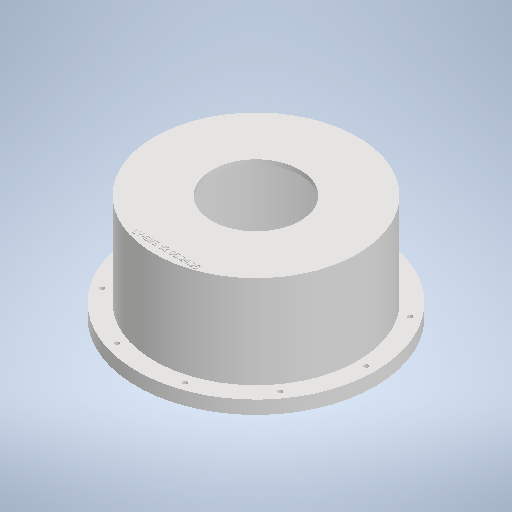
# Autodesk Inventor part: Cylinder Housing
Saved by Autodesk Inventor 2025.2 (Build 292293000, 293)
## iProperties
Created: 2025-06-17
Part Number: Cylinder Housing
Material: Generic
Document SubType Name: Modeling
Designer: mumin
Density: 1 g/cm^3
Appearance: Default
Author: mumin
Autodesk Inventor part; units mm, degrees
note: some values were not read from the file. Chosen so that the rebuilt part matches the saved one: direction of "Hole1".
ref_plane "YZ Plane" through (0, 0, 0) normal (1, 0, 0) x (0, 1, 0)
ref_plane "XZ Plane" through (0, 0, 0) normal (0, 1, 0) x (-1, 0, 0)
ref_plane "XY Plane" through (0, 0, 0) normal (0, 0, 1) x (1, 0, 0)
sketch "Sketch1" plane through (0, 0, 0) normal (0, 1, 0) x (-1, 0, 0)
  circle A0 centre (0, 0) radius 110
  circle A1 centre (0, 0) radius 135
  dimension "d0" = 220
  dimension "d1" = 270
  constraints: 2 centre point, 2 coincident
  measures "d0" diameter of A0
  measures "d1" diameter of A1
extrude "Extrusion1" add sketch "Sketch1" along normal blind 15
sketch "Sketch2" plane through (0, 15, 0) normal (0, 1, 0) x (1, 0, 0)
  circle A0 centre (0, 0) radius 110 projected
  circle A1 centre (0, 0) radius 115
  dimension "d4" = 230
  constraints: 1 centre point, 1 coincident
  measures "d4" diameter of A1
extrude "Extrusion2" add sketch "Sketch2" along normal blind 105
sketch "Sketch3" plane through (0, 120, 0) normal (0, 1, 0) x (1, 0, 0)
  circle A0 centre (0, 0) radius 115 projected
extrude "Extrusion3" add sketch "Sketch3" against normal blind 5
sketch "Sketch4" plane through (0, 120, 0) normal (0, 1, 0) x (1, 0, 0)
  point P0 (0, 0)
  point P1 (0, 0)
  constraints: 1 coincident
hole "Hole1" at (0, 120, 0) direction (0, -1, 0) diameter 100 depth 5
sketch "Sketch5" plane through (0, 15, 0) normal (0, 1, 0) x (1, 0, 0)
  line L0 (-189, 0) -> (189, 0) projected
  point P0 (0, 0)
  point P1 (-125, 0)
  dimension "d23" = 125
  constraints: 1 point on line
  measures "d23" distance of point (0, 0) point (-125, 0)
hole "Hole2" at (-125, 15, 0) direction (0, -1, 0) diameter 5.2 end through all
pattern_circular "Circular Pattern1" count 10 over 360 about axis through (0, -10, 0) along (0, 1, 0) of "Hole2"
sketch "Sketch6" plane through (0, 120, 0) normal (0, 1, 0) x (1, 0, 0)
  line L0 (-34.2404, -100.9913) -> (41.5143, -100.9913) construction
  line L1 (41.5143, -100.9913) -> (41.5143, -112.0132) construction
  line L2 (41.5143, -112.0132) -> (-34.2404, -112.0132) construction
  line L3 (-34.2404, -112.0132) -> (-34.2404, -100.9913) construction
  line L4 (-30.1561, -107.1178) -> (-33.6326, -107.1178)
  line L5 (-33.6326, -107.1178) -> (-33.6326, -101.1178)
  line L6 (-33.6326, -101.1178) -> (-32.8352, -101.1178)
  line L7 (-32.8352, -101.1178) -> (-32.8352, -106.4079)
  line L8 (-32.8352, -106.4079) -> (-30.1561, -106.4079)
  line L9 (-30.1561, -106.4079) -> (-30.1561, -107.1178)
  line L10 (-25.1772, -101.1178) -> (-27.2437, -107.1178)
  line L11 (-27.2437, -107.1178) -> (-28.1043, -107.1178)
  line L12 (-28.1043, -107.1178) -> (-30.1707, -101.1178)
  line L13 (-30.1707, -101.1178) -> (-29.315, -101.1178)
  line L14 (-29.315, -101.1178) -> (-27.6521, -106.1016)
  line L15 (-27.6521, -106.1016) -> (-25.9892, -101.1178)
  line L16 (-25.9892, -101.1178) -> (-25.1772, -101.1178)
  line L17 (-22.5759, -104.8568) -> (-24.8466, -104.8568)
  line L18 (-24.8466, -104.8568) -> (-24.8466, -104.1275)
  line L19 (-24.8466, -104.1275) -> (-22.5759, -104.1275)
  line L20 (-22.5759, -104.1275) -> (-22.5759, -104.8568)
  spline S0 degree 2 poles (-19.0945, -107.2345) (-19.7315, -107.2345) (-20.7866, -106.8455) (-21.1659, -106.4516) knots 0 0 0 1 2 2 2
  spline S1 degree 2 poles (-21.1659, -106.4516) (-21.5451, -106.0529) (-21.9487, -104.8763) (-21.9487, -104.1129) knots 0 0 0 1 2 2 2
  spline S2 degree 2 poles (-21.9487, -104.1129) (-21.9487, -103.3884) (-21.5402, -102.2409) (-21.161, -101.8325) knots 0 0 0 1 2 2 2
  spline S3 degree 2 poles (-21.161, -101.8325) (-20.7963, -101.4387) (-19.7266, -101.0108) (-19.0897, -101.0108) knots 0 0 0 1 2 2 2
  spline S4 degree 2 poles (-19.0897, -101.0108) (-18.7834, -101.0108) (-18.2291, -101.0983) (-17.9762, -101.1761) knots 0 0 0 1 2 2 2
  spline S5 degree 2 poles (-17.9762, -101.1761) (-17.772, -101.2345) (-17.2761, -101.4484) (-17.1253, -101.5262) knots 0 0 0 1 2 2 2
  line L21 (-17.1253, -101.5262) -> (-17.1253, -102.4889)
  line L22 (-17.1253, -102.4889) -> (-17.1934, -102.4889)
  spline S6 degree 2 poles (-17.1934, -102.4889) (-17.3441, -102.3576) (-17.6602, -102.1194) (-17.9519, -101.9832) knots 0 0 0 1 2 2 2
  spline S7 degree 2 poles (-17.9519, -101.9832) (-18.195, -101.8617) (-18.8223, -101.7012) (-19.1821, -101.7012) knots 0 0 0 1 2 2 2
  spline S8 degree 2 poles (-19.1821, -101.7012) (-20.0475, -101.7012) (-21.1172, -103.0043) (-21.1172, -104.0886) knots 0 0 0 1 2 2 2
  spline S9 degree 2 poles (-21.1172, -104.0886) (-21.1172, -104.6915) (-20.8352, -105.5959) (-20.5678, -105.9071) knots 0 0 0 1 2 2 2
  spline S10 degree 2 poles (-20.5678, -105.9071) (-20.3101, -106.2182) (-19.5808, -106.544) (-19.1237, -106.544) knots 0 0 0 1 2 2 2
  spline S11 degree 2 poles (-19.1237, -106.544) (-18.7882, -106.544) (-18.1172, -106.4468) (-17.8887, -106.3495) knots 0 0 0 1 2 2 2
  line L23 (-17.8887, -106.3495) -> (-17.8887, -104.7985)
  line L24 (-17.8887, -104.7985) -> (-19.2793, -104.7985)
  line L25 (-19.2793, -104.7985) -> (-19.2793, -104.0983)
  line L26 (-19.2793, -104.0983) -> (-17.101, -104.0983)
  line L27 (-17.101, -104.0983) -> (-17.101, -106.7191)
  spline S12 degree 2 poles (-17.101, -106.7191) (-17.2518, -106.7871) (-17.7672, -106.9962) (-17.986, -107.0594) knots 0 0 0 1 2 2 2
  spline S13 degree 2 poles (-17.986, -107.0594) (-18.2826, -107.1469) (-18.759, -107.2345) (-19.0945, -107.2345) knots 0 0 0 1 2 2 2
  line L28 (-11.7477, -101.1178) -> (-13.8142, -107.1178)
  line L29 (-13.8142, -107.1178) -> (-14.6748, -107.1178)
  line L30 (-14.6748, -107.1178) -> (-16.7412, -101.1178)
  line L31 (-16.7412, -101.1178) -> (-15.8855, -101.1178)
  line L32 (-15.8855, -101.1178) -> (-14.2226, -106.1016)
  line L33 (-14.2226, -106.1016) -> (-12.5597, -101.1178)
  line L34 (-12.5597, -101.1178) -> (-11.7477, -101.1178)
  spline S14 degree 2 poles (-9.5014, -107.2247) (-10.1529, -107.2247) (-11.067, -106.9524) (-11.4706, -106.758) knots 0 0 0 1 2 2 2
  line L35 (-11.4706, -106.758) -> (-11.4706, -105.7563)
  line L36 (-11.4706, -105.7563) -> (-11.4122, -105.7563)
  spline S15 degree 2 poles (-11.4122, -105.7563) (-11.0184, -106.1259) (-10.0216, -106.5343) (-9.5597, -106.5343) knots 0 0 0 1 2 2 2
  spline S16 degree 2 poles (-9.5597, -106.5343) (-8.8984, -106.5343) (-8.2226, -105.9849) (-8.2226, -105.5327) knots 0 0 0 1 2 2 2
  spline S17 degree 2 poles (-8.2226, -105.5327) (-8.2226, -105.1729) (-8.5775, -104.7255) (-8.9616, -104.6137) knots 0 0 0 1 2 2 2
  spline S18 degree 2 poles (-8.9616, -104.6137) (-9.2388, -104.5359) (-9.7007, -104.4289) (-10.0459, -104.3414) knots 0 0 0 1 2 2 2
  spline S19 degree 2 poles (-10.0459, -104.3414) (-10.3571, -104.2588) (-10.8482, -104.0108) (-11.0378, -103.8114) knots 0 0 0 1 2 2 2
  spline S20 degree 2 poles (-11.0378, -103.8114) (-11.2226, -103.6121) (-11.4268, -103.0772) (-11.4268, -102.7272) knots 0 0 0 1 2 2 2
  spline S21 degree 2 poles (-11.4268, -102.7272) (-11.4268, -101.9978) (-10.289, -101.0108) (-9.409, -101.0108) knots 0 0 0 1 2 2 2
  spline S22 degree 2 poles (-9.409, -101.0108) (-8.9033, -101.0108) (-8.0086, -101.2101) (-7.6245, -101.3998) knots 0 0 0 1 2 2 2
  line L37 (-7.6245, -101.3998) -> (-7.6245, -102.3528)
  line L38 (-7.6245, -102.3528) -> (-7.6829, -102.3528)
  spline S23 degree 2 poles (-7.6829, -102.3528) (-7.9697, -102.0902) (-8.8644, -101.7012) (-9.3555, -101.7012) knots 0 0 0 1 2 2 2
  spline S24 degree 2 poles (-9.3555, -101.7012) (-9.9098, -101.7012) (-10.5954, -102.2215) (-10.5954, -102.6445) knots 0 0 0 1 2 2 2
  spline S25 degree 2 poles (-10.5954, -102.6445) (-10.5954, -103.0238) (-10.1918, -103.4759) (-9.8125, -103.5781) knots 0 0 0 1 2 2 2
  spline S26 degree 2 poles (-9.8125, -103.5781) (-9.5597, -103.6461) (-8.8255, -103.8212) (-8.5824, -103.8941) knots 0 0 0 1 2 2 2
  spline S27 degree 2 poles (-8.5824, -103.8941) (-7.9649, -104.0837) (-7.3911, -104.8471) (-7.3911, -105.4063) knots 0 0 0 1 2 2 2
  spline S28 degree 2 poles (-7.3911, -105.4063) (-7.3911, -105.7612) (-7.678, -106.4419) (-7.9357, -106.6802) knots 0 0 0 1 2 2 2
  spline S29 degree 2 poles (-7.9357, -106.6802) (-8.2226, -106.9427) (-8.9519, -107.2247) (-9.5014, -107.2247) knots 0 0 0 1 2 2 2
  line L39 (0.3495, -101.1178) -> (-1.7169, -107.1178)
  line L40 (-1.7169, -107.1178) -> (-2.5775, -107.1178)
  line L41 (-2.5775, -107.1178) -> (-4.644, -101.1178)
  line L42 (-4.644, -101.1178) -> (-3.7882, -101.1178)
  line L43 (-3.7882, -101.1178) -> (-2.1253, -106.1016)
  line L44 (-2.1253, -106.1016) -> (-0.4625, -101.1178)
  line L45 (-0.4625, -101.1178) -> (0.3495, -101.1178)
  spline S30 degree 2 poles (2.3722, -101.6866) (2.1534, -101.6866) (1.7207, -101.7936) (1.5116, -101.8763) knots 0 0 0 1 2 2 2
  spline S31 degree 2 poles (1.5116, -101.8763) (1.3171, -101.9589) (1.0303, -102.134) (0.9184, -102.2118) knots 0 0 0 1 2 2 2
  line L46 (0.9184, -102.2118) -> (0.8698, -102.2118)
  line L47 (0.8698, -102.2118) -> (0.8698, -101.3609)
  spline S32 degree 2 poles (0.8698, -101.3609) (1.1324, -101.2199) (2.0319, -100.9913) (2.4354, -100.9913) knots 0 0 0 1 2 2 2
  spline S33 degree 2 poles (2.4354, -100.9913) (2.8439, -100.9913) (3.4516, -101.1567) (3.6996, -101.3317) knots 0 0 0 1 2 2 2
  spline S34 degree 2 poles (3.6996, -101.3317) (3.9622, -101.5213) (4.2345, -102.0708) (4.2345, -102.4403) knots 0 0 0 1 2 2 2
  spline S35 degree 2 poles (4.2345, -102.4403) (4.2345, -102.9362) (3.5829, -103.685) (3.1259, -103.7823) knots 0 0 0 1 2 2 2
  line L48 (3.1259, -103.7823) -> (3.1259, -103.8406)
  spline S36 degree 2 poles (3.1259, -103.8406) (3.3155, -103.8795) (3.7482, -104.0546) (3.933, -104.2296) knots 0 0 0 1 2 2 2
  spline S37 degree 2 poles (3.933, -104.2296) (4.1178, -104.3998) (4.3512, -104.9443) (4.3512, -105.3382) knots 0 0 0 1 2 2 2
  spline S38 degree 2 poles (4.3512, -105.3382) (4.3512, -105.7418) (4.074, -106.4273) (3.8212, -106.6899) knots 0 0 0 1 2 2 2
  spline S39 degree 2 poles (3.8212, -106.6899) (3.5586, -106.9622) (2.8147, -107.2442) (2.3431, -107.2442) knots 0 0 0 1 2 2 2
  spline S40 degree 2 poles (2.3431, -107.2442) (1.8909, -107.2442) (1.0059, -107.0254) (0.7045, -106.8747) knots 0 0 0 1 2 2 2
  line L49 (0.7045, -106.8747) -> (0.7045, -106.0238)
  line L50 (0.7045, -106.0238) -> (0.7628, -106.0238)
  spline S41 degree 2 poles (0.7628, -106.0238) (1.0157, -106.2085) (1.8714, -106.5489) (2.2944, -106.5489) knots 0 0 0 1 2 2 2
  spline S42 degree 2 poles (2.2944, -106.5489) (2.5424, -106.5489) (3.0384, -106.3933) (3.2037, -106.2134) knots 0 0 0 1 2 2 2
  spline S43 degree 2 poles (3.2037, -106.2134) (3.3641, -106.0335) (3.5343, -105.6056) (3.5343, -105.2798) knots 0 0 0 1 2 2 2
  spline S44 degree 2 poles (3.5343, -105.2798) (3.5343, -104.9541) (3.3447, -104.5311) (3.1745, -104.4095) knots 0 0 0 1 2 2 2
  spline S45 degree 2 poles (3.1745, -104.4095) (3.0043, -104.2879) (2.5424, -104.1956) (2.2701, -104.1956) knots 0 0 0 1 2 2 2
  line L51 (2.2701, -104.1956) -> (1.9298, -104.1956)
  line L52 (1.9298, -104.1956) -> (1.9298, -103.5294)
  line L53 (1.9298, -103.5294) -> (2.1972, -103.5294)
  spline S46 degree 2 poles (2.1972, -103.5294) (2.7369, -103.5294) (3.4176, -103.014) (3.4176, -102.5229) knots 0 0 0 1 2 2 2
  spline S47 degree 2 poles (3.4176, -102.5229) (3.4176, -102.2944) (3.2426, -101.9687) (3.1016, -101.8714) knots 0 0 0 1 2 2 2
  spline S48 degree 2 poles (3.1016, -101.8714) (2.9508, -101.7693) (2.5813, -101.6866) (2.3722, -101.6866) knots 0 0 0 1 2 2 2
  spline S49 degree 2 poles (11.5667, -104.1178) (11.5667, -105.732) (10.6283, -107.2442) (9.651, -107.2442) knots 0 0 0 1 2 2 2
  spline S50 degree 2 poles (9.651, -107.2442) (8.6591, -107.2442) (7.7304, -105.7029) (7.7304, -104.1226) knots 0 0 0 1 2 2 2
  spline S51 degree 2 poles (7.7304, -104.1226) (7.7304, -102.4986) (8.6688, -100.9962) (9.651, -100.9962) knots 0 0 0 1 2 2 2
  spline S52 degree 2 poles (9.651, -100.9962) (10.638, -100.9962) (11.5667, -102.5521) (11.5667, -104.1178) knots 0 0 0 1 2 2 2
  spline S53 degree 2 poles (10.5359, -105.946) (10.6526, -105.6494) (10.7499, -104.7353) (10.7499, -104.1178) knots 0 0 0 1 2 2 2
  spline S54 degree 2 poles (10.7499, -104.1178) (10.7499, -103.5003) (10.6526, -102.591) (10.5311, -102.2847) knots 0 0 0 1 2 2 2
  spline S55 degree 2 poles (10.5311, -102.2847) (10.4095, -101.9784) (9.9865, -101.6623) (9.651, -101.6623) knots 0 0 0 1 2 2 2
  spline S56 degree 2 poles (9.651, -101.6623) (9.3155, -101.6623) (8.8828, -101.9784) (8.7563, -102.2944) knots 0 0 0 1 2 2 2
  spline S57 degree 2 poles (8.7563, -102.2944) (8.6348, -102.6007) (8.5473, -103.5343) (8.5473, -104.1226) knots 0 0 0 1 2 2 2
  spline S58 degree 2 poles (8.5473, -104.1226) (8.5473, -104.7547) (8.6251, -105.6007) (8.7515, -105.9314) knots 0 0 0 1 2 2 2
  spline S59 degree 2 poles (8.7515, -105.9314) (8.8682, -106.2426) (9.3009, -106.5781) (9.651, -106.5781) knots 0 0 0 1 2 2 2
  spline S60 degree 2 poles (9.651, -106.5781) (9.9816, -106.5781) (10.4144, -106.262) (10.5359, -105.946) knots 0 0 0 1 2 2 2
  spline S61 degree 2 poles (16.1275, -105.1729) (16.1275, -105.6348) (15.8212, -106.4176) (15.5635, -106.6802) knots 0 0 0 1 2 2 2
  spline S62 degree 2 poles (15.5635, -106.6802) (15.2961, -106.9573) (14.6251, -107.2442) (14.2215, -107.2442) knots 0 0 0 1 2 2 2
  spline S63 degree 2 poles (14.2215, -107.2442) (13.8179, -107.2442) (13.1518, -106.9719) (12.899, -106.6996) knots 0 0 0 1 2 2 2
  spline S64 degree 2 poles (12.899, -106.6996) (12.5878, -106.3738) (12.2377, -105.2798) (12.2377, -104.4824) knots 0 0 0 1 2 2 2
  spline S65 degree 2 poles (12.2377, -104.4824) (12.2377, -103.6996) (12.5586, -102.4403) (12.8941, -101.9735) knots 0 0 0 1 2 2 2
  spline S66 degree 2 poles (12.8941, -101.9735) (13.2199, -101.5165) (14.2507, -101.0059) (14.9265, -101.0059) knots 0 0 0 1 2 2 2
  spline S67 degree 2 poles (14.9265, -101.0059) (15.1259, -101.0059) (15.476, -101.0448) (15.6072, -101.0886) knots 0 0 0 1 2 2 2
  line L54 (15.6072, -101.0886) -> (15.6072, -101.8617)
  line L55 (15.6072, -101.8617) -> (15.5732, -101.8617)
  spline S68 degree 2 poles (15.5732, -101.8617) (15.4614, -101.8033) (15.0529, -101.7012) (14.8196, -101.7012) knots 0 0 0 1 2 2 2
  spline S69 degree 2 poles (14.8196, -101.7012) (14.0708, -101.7012) (13.1518, -102.7126) (13.0643, -103.7045) knots 0 0 0 1 2 2 2
  spline S70 degree 2 poles (13.0643, -103.7045) (13.3512, -103.5051) (13.9541, -103.2863) (14.3139, -103.2863) knots 0 0 0 1 2 2 2
  spline S71 degree 2 poles (14.3139, -103.2863) (14.664, -103.2863) (15.1891, -103.4273) (15.476, -103.6413) knots 0 0 0 1 2 2 2
  spline S72 degree 2 poles (15.476, -103.6413) (15.8066, -103.8892) (16.1275, -104.6575) (16.1275, -105.1729) knots 0 0 0 1 2 2 2
  spline S73 degree 2 poles (15.3106, -105.2069) (15.3106, -104.8374) (15.1162, -104.3366) (14.9022, -104.1615) knots 0 0 0 1 2 2 2
  spline S74 degree 2 poles (14.9022, -104.1615) (14.7418, -104.0351) (14.3431, -103.9524) (14.134, -103.9524) knots 0 0 0 1 2 2 2
  spline S75 degree 2 poles (14.134, -103.9524) (13.852, -103.9524) (13.322, -104.1226) (13.0643, -104.2831) knots 0 0 0 1 2 2 2
  spline S76 degree 2 poles (13.0643, -104.2831) (13.0594, -104.3706) (13.0497, -104.5359) (13.0497, -104.6623) knots 0 0 0 1 2 2 2
  spline S77 degree 2 poles (13.0497, -104.6623) (13.0497, -105.2847) (13.2928, -106.0481) (13.4776, -106.2474) knots 0 0 0 1 2 2 2
  spline S78 degree 2 poles (13.4776, -106.2474) (13.6478, -106.4371) (14.0173, -106.5878) (14.2264, -106.5878) knots 0 0 0 1 2 2 2
  spline S79 degree 2 poles (14.2264, -106.5878) (14.7126, -106.5878) (15.3106, -105.8973) (15.3106, -105.2069) knots 0 0 0 1 2 2 2
  line L56 (18.1259, -107.1178) -> (17.1632, -107.1178)
  line L57 (17.1632, -107.1178) -> (17.1632, -105.9703)
  line L58 (17.1632, -105.9703) -> (18.1259, -105.9703)
  line L59 (18.1259, -105.9703) -> (18.1259, -107.1178)
  line L60 (23.0367, -107.1178) -> (19.3366, -107.1178)
  line L61 (19.3366, -107.1178) -> (19.3366, -106.2669)
  spline S80 degree 2 poles (19.3366, -106.2669) (19.7353, -105.8925) (20.4452, -105.1972) (20.7855, -104.8228) knots 0 0 0 1 2 2 2
  spline S81 degree 2 poles (20.7855, -104.8228) (21.4711, -104.0691) (21.9719, -103.1648) (21.9719, -102.6834) knots 0 0 0 1 2 2 2
  spline S82 degree 2 poles (21.9719, -102.6834) (21.9719, -102.4306) (21.8163, -102.0513) (21.6753, -101.9298) knots 0 0 0 1 2 2 2
  spline S83 degree 2 poles (21.6753, -101.9298) (21.5343, -101.8082) (21.1648, -101.6866) (20.9411, -101.6866) knots 0 0 0 1 2 2 2
  spline S84 degree 2 poles (20.9411, -101.6866) (20.7272, -101.6866) (20.2896, -101.7936) (20.0902, -101.8763) knots 0 0 0 1 2 2 2
  spline S85 degree 2 poles (20.0902, -101.8763) (19.92, -101.9443) (19.604, -102.1388) (19.5068, -102.2069) knots 0 0 0 1 2 2 2
  line L62 (19.5068, -102.2069) -> (19.463, -102.2069)
  line L63 (19.463, -102.2069) -> (19.463, -101.3512)
  spline S86 degree 2 poles (19.463, -101.3512) (19.711, -101.2296) (20.6008, -100.9913) (20.9995, -100.9913) knots 0 0 0 1 2 2 2
  spline S87 degree 2 poles (20.9995, -100.9913) (21.8406, -100.9913) (22.7888, -101.8811) (22.7888, -102.6396) knots 0 0 0 1 2 2 2
  spline S88 degree 2 poles (22.7888, -102.6396) (22.7888, -102.9946) (22.6234, -103.5878) (22.4776, -103.8406) knots 0 0 0 1 2 2 2
  spline S89 degree 2 poles (22.4776, -103.8406) (22.3317, -104.1032) (21.9087, -104.6186) (21.6753, -104.8665) knots 0 0 0 1 2 2 2
  spline S90 degree 2 poles (21.6753, -104.8665) (21.2961, -105.2798) (20.3674, -106.1648) (20.0902, -106.4225) knots 0 0 0 1 2 2 2
  line L64 (20.0902, -106.4225) -> (23.0367, -106.4225)
  line L65 (23.0367, -106.4225) -> (23.0367, -107.1178)
  line L66 (27.6996, -105.0562) -> (26.9849, -105.0562)
  line L67 (26.9849, -105.0562) -> (26.9849, -107.1178)
  line L68 (26.9849, -107.1178) -> (26.2118, -107.1178)
  line L69 (26.2118, -107.1178) -> (26.2118, -105.0562)
  line L70 (26.2118, -105.0562) -> (23.5619, -105.0562)
  line L71 (23.5619, -105.0562) -> (23.5619, -104.2101)
  line L72 (23.5619, -104.2101) -> (26.2458, -101.1178)
  line L73 (26.2458, -101.1178) -> (26.9849, -101.1178)
  line L74 (26.9849, -101.1178) -> (26.9849, -104.4095)
  line L75 (26.9849, -104.4095) -> (27.6996, -104.4095)
  line L76 (27.6996, -104.4095) -> (27.6996, -105.0562)
  line L77 (26.2118, -104.4095) -> (26.2118, -102.0659)
  line L78 (26.2118, -102.0659) -> (24.194, -104.4095)
  line L79 (24.194, -104.4095) -> (26.2118, -104.4095)
  line L80 (29.6299, -107.1178) -> (28.6672, -107.1178)
  line L81 (28.6672, -107.1178) -> (28.6672, -105.9703)
  line L82 (28.6672, -105.9703) -> (29.6299, -105.9703)
  line L83 (29.6299, -105.9703) -> (29.6299, -107.1178)
  line L84 (34.5408, -107.1178) -> (30.8406, -107.1178)
  line L85 (30.8406, -107.1178) -> (30.8406, -106.2669)
  spline S91 degree 2 poles (30.8406, -106.2669) (31.2393, -105.8925) (31.9492, -105.1972) (32.2896, -104.8228) knots 0 0 0 1 2 2 2
  spline S92 degree 2 poles (32.2896, -104.8228) (32.9752, -104.0691) (33.476, -103.1648) (33.476, -102.6834) knots 0 0 0 1 2 2 2
  spline S93 degree 2 poles (33.476, -102.6834) (33.476, -102.4306) (33.3204, -102.0513) (33.1794, -101.9298) knots 0 0 0 1 2 2 2
  spline S94 degree 2 poles (33.1794, -101.9298) (33.0384, -101.8082) (32.6688, -101.6866) (32.4452, -101.6866) knots 0 0 0 1 2 2 2
  spline S95 degree 2 poles (32.4452, -101.6866) (32.2312, -101.6866) (31.7936, -101.7936) (31.5943, -101.8763) knots 0 0 0 1 2 2 2
  spline S96 degree 2 poles (31.5943, -101.8763) (31.4241, -101.9443) (31.1081, -102.1388) (31.0108, -102.2069) knots 0 0 0 1 2 2 2
  line L86 (31.0108, -102.2069) -> (30.967, -102.2069)
  line L87 (30.967, -102.2069) -> (30.967, -101.3512)
  spline S97 degree 2 poles (30.967, -101.3512) (31.215, -101.2296) (32.1048, -100.9913) (32.5035, -100.9913) knots 0 0 0 1 2 2 2
  spline S98 degree 2 poles (32.5035, -100.9913) (33.3447, -100.9913) (34.2928, -101.8811) (34.2928, -102.6396) knots 0 0 0 1 2 2 2
  spline S99 degree 2 poles (34.2928, -102.6396) (34.2928, -102.9946) (34.1275, -103.5878) (33.9816, -103.8406) knots 0 0 0 1 2 2 2
  spline S100 degree 2 poles (33.9816, -103.8406) (33.8358, -104.1032) (33.4128, -104.6186) (33.1794, -104.8665) knots 0 0 0 1 2 2 2
  spline S101 degree 2 poles (33.1794, -104.8665) (32.8001, -105.2798) (31.8714, -106.1648) (31.5943, -106.4225) knots 0 0 0 1 2 2 2
  line L88 (31.5943, -106.4225) -> (34.5408, -106.4225)
  line L89 (34.5408, -106.4225) -> (34.5408, -107.1178)
  spline S102 degree 2 poles (38.98, -105.2118) (38.98, -105.6445) (38.7029, -106.3836) (38.45, -106.6559) knots 0 0 0 1 2 2 2
  spline S103 degree 2 poles (38.45, -106.6559) (38.1972, -106.9281) (37.4435, -107.2442) (36.9768, -107.2442) knots 0 0 0 1 2 2 2
  spline S104 degree 2 poles (36.9768, -107.2442) (36.5489, -107.2442) (35.7126, -107.0546) (35.4063, -106.9038) knots 0 0 0 1 2 2 2
  line L90 (35.4063, -106.9038) -> (35.4063, -106.0529)
  line L91 (35.4063, -106.0529) -> (35.4646, -106.0529)
  spline S105 degree 2 poles (35.4646, -106.0529) (35.557, -106.121) (35.9022, -106.296) (36.1113, -106.3738) knots 0 0 0 1 2 2 2
  spline S106 degree 2 poles (36.1113, -106.3738) (36.3495, -106.4565) (36.7434, -106.5489) (36.9914, -106.5489) knots 0 0 0 1 2 2 2
  spline S107 degree 2 poles (36.9914, -106.5489) (37.2345, -106.5489) (37.6915, -106.3738) (37.8568, -106.1842) knots 0 0 0 1 2 2 2
  spline S108 degree 2 poles (37.8568, -106.1842) (38.0076, -106.0043) (38.1632, -105.5278) (38.1632, -105.2069) knots 0 0 0 1 2 2 2
  spline S109 degree 2 poles (38.1632, -105.2069) (38.1632, -104.886) (37.9881, -104.4776) (37.8228, -104.3414) knots 0 0 0 1 2 2 2
  spline S110 degree 2 poles (37.8228, -104.3414) (37.6526, -104.1907) (37.1469, -104.0643) (36.8406, -104.0643) knots 0 0 0 1 2 2 2
  spline S111 degree 2 poles (36.8406, -104.0643) (36.51, -104.0643) (35.8536, -104.1664) (35.6542, -104.2101) knots 0 0 0 1 2 2 2
  line L92 (35.6542, -104.2101) -> (35.6542, -101.1178)
  line L93 (35.6542, -101.1178) -> (38.946, -101.1178)
  line L94 (38.946, -101.1178) -> (38.946, -101.8228)
  line L95 (38.946, -101.8228) -> (36.4273, -101.8228)
  line L96 (36.4273, -101.8228) -> (36.4273, -103.4225)
  spline S112 degree 2 poles (36.4273, -103.4225) (36.5732, -103.403) (36.8552, -103.3884) (36.9719, -103.3884) knots 0 0 0 1 2 2 2
  spline S113 degree 2 poles (36.9719, -103.3884) (37.4338, -103.3884) (38.0708, -103.5392) (38.3625, -103.7628) knots 0 0 0 1 2 2 2
  spline S114 degree 2 poles (38.3625, -103.7628) (38.6591, -103.9865) (38.98, -104.6672) (38.98, -105.2118) knots 0 0 0 1 2 2 2
  point P0 (0, 0)
  constraints: 2 other
extrude "Extrusion4" add sketch "Sketch6" along normal blind 1
body "Solid1"
